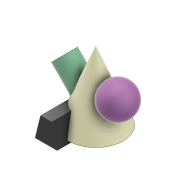
# Autodesk Inventor part: Деталь1
Saved by Autodesk Inventor 2021.2 (Build 252289000, 289)
## iProperties
Created: 2023-10-19
Part Number: Деталь1
Material: Типовые
Document SubType Name: Modeling
Designer: User
Density: 1 g/cm^3
Appearance: По умолчанию
Mass: 624.878 g
Surface Area: 652.499 cm^2
Volume: 624.878 cm^3
Author: User
Autodesk Inventor part; units mm, degrees
ref_plane "YZ Plane" through (0, 0, 0) normal (1, 0, 0) x (0, 1, 0)
ref_plane "XZ Plane" through (0, 0, 0) normal (0, 1, 0) x (-1, 0, 0)
ref_plane "XY Plane" through (0, 0, 0) normal (0, 0, 1) x (1, 0, 0)
sketch "Эскиз2" plane through (0, 0, 0) normal (0, 0, 1) x (1, 0, 0)
  line L0 (0, 0) -> (50, 0)
  line L1 (0, 0) -> (0, 125)
  line L2 (0, 125) -> (50, 0)
  dimension "d4" = 50
  dimension "d5" = 125
  constraints: 6 end point, 1 horizontal, 1 vertical
  measures "d4" distance of L0.start L0.end
  measures "d5" distance of L0.start L1.end
revolve "Вращение2" add sketch "Эскиз2" angle 360 about axis through (0, 0, 0) along (0, 1, 0)
sketch "Эскиз3" plane through (0, 0, 0) normal (0, 0, 1) x (1, 0, 0)
  line L0 (0, -5) -> (-40, -5)
  line L1 (-10, 35) -> (0, -5)
  line L2 (-10, 35) -> (-30, 35)
  line L3 (-50, 0) -> (50, 0) projected
  line L4 (-30, 35) -> (-40, -5)
  point P0 (0, 0)
  dimension "d7" = 40
  dimension "d8" = 20
  constraints: 8 end point, 1 horizontal, 1 parallel
  measures "d7" distance of L0.start L0.end
  measures "d8" distance of L1.start L2.end
extrude "Выдавливание1" add sketch "Эскиз3" along normal blind 70 separate body
sketch "Эскиз4" plane through (0, 0, 0) normal (0, 0, 1) x (1, 0, 0)
  circle A0 centre (40, 60) radius 30
  line L0 (40, 90) -> (40, 30)
  point P0 (0, 0)
  dimension "d11" = 60
  constraints: 2 end point, 2 point on circle, 1 centre point, 1 vertical
  measures "d11" diameter of A0
revolve "Вращение3" add sketch "Эскиз4" angle 360 about axis through (40, 90, 0) along (0, -1, 0) separate body picked at (52.2687, 66.2349) contours A0 L0
sketch "Эскиз5" plane through (0, 0, 0) normal (0, 0, 1) x (1, 0, 0)
  line L0 (0, 26) -> (-56.5685, 82.5685)
  line L1 (-56.5685, 82.5685) -> (-42.4264, 96.7107)
  line L2 (-42.4264, 96.7107) -> (14.1421, 40.1421)
  line L3 (14.1421, 40.1421) -> (0, 26)
  line L4 (0, 26) -> (80, 26) construction
  point P0 (0, 0)
  dimension "d13" = 80
  dimension "d14" = 135
  dimension "d15" = 20
  constraints: 10 end point, 2 parallel, 1 equal length, 1 horizontal, 1 perpendicular
  measures "d13" distance of L0.start L0.end
  measures "d14" angle of L4 L0
  measures "d15" distance of L0.end L1.end
revolve "Вращение4" add sketch "Эскиз5" angle 360 about axis through (0, 26, 0) along (-0.7071, 0.7071, 0) separate body
